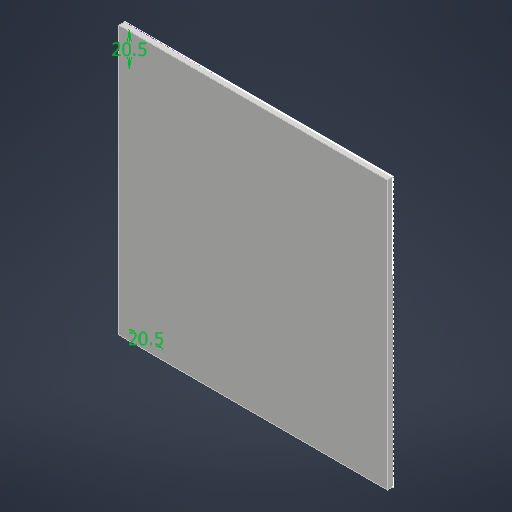
# Autodesk Inventor part: Marble Maze Template
Saved by Autodesk Inventor 2026.1 (Build 301233000, 233)
## iProperties
Created: 2021-01-22
Part Number: Marble Maze Template
Material: Generic
Document SubType Name: Modeling
Designer: ScottSt
Density: 1 g/cm^3
Appearance: Default
Author: ScottSt
Autodesk Inventor part; units mm, degrees
ref_plane "YZ Plane" through (0, 0, 0) normal (1, 0, 0) x (0, 1, 0)
ref_plane "XZ Plane" through (0, 0, 0) normal (0, 1, 0) x (-1, 0, 0)
ref_plane "XY Plane" through (0, 0, 0) normal (0, 0, 1) x (1, 0, 0)
sketch "Sketch1" plane through (0, 0, 0) normal (0, 1, 0) x (-1, 0, 0)
  line L0 (83.5, -83.5) -> (-83.5, -83.5)
  line L1 (-83.5, -83.5) -> (-83.5, 83.5)
  line L2 (-83.5, 83.5) -> (83.5, 83.5)
  line L3 (83.5, 83.5) -> (83.5, -83.5)
  line L4 (83.5, -83.5) -> (-83.5, 83.5) construction
  line L5 (-83.5, -83.5) -> (83.5, 83.5) construction
  point P0 (0, 0)
  dimension "d6" = 167
  dimension "d7" = 167
  constraints: 12 end point, 2 midpoint, 2 parallel, 1 horizontal, 1 perpendicular
  measures "d6" distance of L1.end L2.end
  measures "d7" distance of L0.end L1.end
extrude "Extrusion3" add sketch "Sketch1" along normal blind 3.5
sketch "Maze Layout" plane through (0, 3.5, 0) normal (0, 1, 0) x (1, 0, 0)
  line L0 (83.5, 83.5) -> (-83.5, 83.5) construction
  line L1 (83.5, -83.5) -> (83.5, 83.5) construction
  line L2 (-83.5, 83.5) -> (83.5, 83.5) construction
  line L3 (83.5, 83.5) -> (83.5, -83.5) construction
  line L4 (-80.5, -80.5) -> (80.5, -80.5) construction
  line L5 (80.5, -80.5) -> (80.5, 80.5) construction
  line L6 (80.5, 80.5) -> (-80.5, 80.5) construction
  line L7 (-80.5, 80.5) -> (-80.5, -80.5) construction
  line L8 (-80.5, -80.5) -> (-83.5, -80.5) construction
  line L9 (-83.5, -80.5) -> (-80.5, -80.5) construction
  line L10 (-80.5, -80.5) -> (-80.5, -83.5) construction
  line L11 (-83.5, -80.5) -> (-83.5, 80.5) construction
  line L12 (-83.5, 83.5) -> (-83.5, -83.5) construction
  line L13 (-83.5, 80.5) -> (-80.5, 80.5) construction
  line L14 (-60, 80.5) -> (-60, -80.5) construction
  line L15 (-63, -80.5) -> (-63, 80.5) construction
  line L16 (-63, 80.5) -> (-60, 80.5) construction
  line L17 (-60, -80.5) -> (-63, -80.5) construction
  line L18 (-39.5, 80.5) -> (-39.5, -80.5) construction
  line L19 (-42.5, -80.5) -> (-42.5, 80.5) construction
  line L20 (-42.5, 80.5) -> (-39.5, 80.5) construction
  line L21 (-39.5, -80.5) -> (-42.5, -80.5) construction
  line L22 (-19, 80.5) -> (-19, -80.5) construction
  line L23 (-22, -80.5) -> (-22, 80.5) construction
  line L24 (-22, 80.5) -> (-19, 80.5) construction
  line L25 (-19, -80.5) -> (-22, -80.5) construction
  line L26 (1.5, 80.5) -> (1.5, -80.5) construction
  line L27 (-1.5, -80.5) -> (-1.5, 80.5) construction
  line L28 (-1.5, 80.5) -> (1.5, 80.5) construction
  line L29 (1.5, -80.5) -> (-1.5, -80.5) construction
  line L30 (22, 80.5) -> (22, -80.5) construction
  line L31 (19, -80.5) -> (19, 80.5) construction
  line L32 (19, 80.5) -> (22, 80.5) construction
  line L33 (22, -80.5) -> (19, -80.5) construction
  line L34 (42.5, 80.5) -> (42.5, -80.5) construction
  line L35 (39.5, -80.5) -> (39.5, 80.5) construction
  line L36 (39.5, 80.5) -> (42.5, 80.5) construction
  line L37 (42.5, -80.5) -> (39.5, -80.5) construction
  line L38 (63, 80.5) -> (63, -80.5) construction
  line L39 (60, -80.5) -> (60, 80.5) construction
  line L40 (60, 80.5) -> (63, 80.5) construction
  line L41 (63, -80.5) -> (60, -80.5) construction
  line L42 (-80.5, -83.5) -> (80.5, -83.5) construction
  line L43 (80.5, -83.5) -> (80.5, -80.5) construction
  line L44 (-80.5, -60) -> (-80.5, -63) construction
  line L45 (-80.5, -60) -> (80.5, -60) construction
  line L46 (-80.5, -63) -> (80.5, -63) construction
  line L47 (80.5, -63) -> (80.5, -60) construction
  line L48 (-80.5, -39.5) -> (-80.5, -42.5) construction
  line L49 (-80.5, -39.5) -> (80.5, -39.5) construction
  line L50 (-80.5, -42.5) -> (80.5, -42.5) construction
  line L51 (80.5, -42.5) -> (80.5, -39.5) construction
  line L52 (-80.5, -19) -> (-80.5, -22) construction
  line L53 (-80.5, -19) -> (80.5, -19) construction
  line L54 (-80.5, -22) -> (80.5, -22) construction
  line L55 (80.5, -22) -> (80.5, -19) construction
  line L56 (-80.5, 1.5) -> (-80.5, -1.5) construction
  line L57 (-80.5, 1.5) -> (80.5, 1.5) construction
  line L58 (-80.5, -1.5) -> (80.5, -1.5) construction
  line L59 (80.5, -1.5) -> (80.5, 1.5) construction
  line L60 (-80.5, 22) -> (-80.5, 19) construction
  line L61 (-80.5, 22) -> (80.5, 22) construction
  line L62 (-80.5, 19) -> (80.5, 19) construction
  line L63 (80.5, 19) -> (80.5, 22) construction
  line L64 (-80.5, 42.5) -> (-80.5, 39.5) construction
  line L65 (-80.5, 42.5) -> (80.5, 42.5) construction
  line L66 (-80.5, 39.5) -> (80.5, 39.5) construction
  line L67 (80.5, 39.5) -> (80.5, 42.5) construction
  line L68 (-80.5, 63) -> (-80.5, 60) construction
  line L69 (-80.5, 63) -> (80.5, 63) construction
  line L70 (-80.5, 60) -> (80.5, 60) construction
  line L71 (80.5, 60) -> (80.5, 63) construction
  line L72 (42.5, 80.5) -> (39.5, 80.5)
  line L73 (22, 80.5) -> (19, 80.5)
  line L74 (-22, 80.5) -> (-19, 80.5)
  line L75 (-80.5, 60) -> (-80.5, 63)
  line L76 (80.5, 60) -> (80.5, 63)
  line L77 (80.5, 1.5) -> (80.5, -1.5)
  line L78 (63, -80.5) -> (60, -80.5)
  line L79 (22, -80.5) -> (19, -80.5)
  line L80 (-39.5, -80.5) -> (-42.5, -80.5)
  line L81 (-80.5, -60) -> (-80.5, -63)
  line L82 (-80.5, -19) -> (-80.5, -22)
  line L83 (83.5, -83.5) -> (-83.5, -83.5)
  line L84 (-83.5, -83.5) -> (-83.5, 83.5)
  line L85 (-83.5, 83.5) -> (83.5, 83.5)
  line L86 (83.5, 83.5) -> (83.5, -83.5)
  line L87 (-80.5, 80.5) -> (80.5, 80.5)
  line L88 (80.5, 80.5) -> (80.5, -80.5)
  line L89 (80.5, -80.5) -> (-80.5, -80.5)
  line L90 (-80.5, -80.5) -> (-80.5, 80.5)
  dimension "d25" = 20.5
  dimension "d32" = 20.5
  constraints: 176 end point, 10 horizontal, 7 equal length, 5 perpendicular, 2 point on line, 1 vertical, 113 other
  measures "d25" distance of L6.end L14.start
  measures "d32" distance of L4.start L44.start
body "Solid3"
